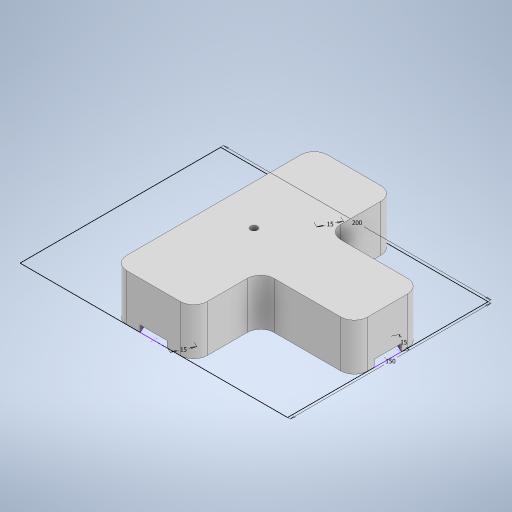
# Autodesk Inventor part: Area mv
Saved by Autodesk Inventor 2024 (Build 280153000, 153)
## iProperties
Created: 2024-03-01
Part Number: Area mv
Material: Generic
Document SubType Name: Modeling
Designer: laura
Density: 1 g/cm^3
Appearance: Default
Author: laura
Autodesk Inventor part; units mm, degrees
ref_plane "YZ Plane" through (0, 0, 0) normal (1, 0, 0) x (0, 1, 0)
ref_plane "XZ Plane" through (0, 0, 0) normal (0, 1, 0) x (-1, 0, 0)
ref_plane "XY Plane" through (0, 0, 0) normal (0, 0, 1) x (1, 0, 0)
sketch "Sketch1" plane through (0, 0, 0) normal (0, 1, 0) x (-1, 0, 0)
  line L0 (0, 0) -> (-200, 0)
  line L1 (-200, 0) -> (-200, -150)
  line L2 (-200, -150) -> (0, -150)
  line L3 (0, -150) -> (0, 0)
  line L4 (-109.8726, -150) -> (-90.1274, -150)
  line L5 (-200, -85.1274) -> (-200, -64.8726)
  line L6 (-186.0054, -60.2304) -> (-186.0054, -75)
  line L7 (-200, -64.8726) -> (-187.7125, -59.1428)
  arc A0 (-186.0054, -60.2304) -> (-187.7125, -59.1428) centre (-187.2054, -60.2304) ccw
  line L8 (-186.0054, -75) -> (-186.0054, -89.7696)
  line L9 (-199.8, -85) -> (-186.3697, -85) construction
  arc A1 (-187.7125, -90.8572) -> (-186.0054, -89.7696) centre (-187.2054, -89.7696) ccw
  line L10 (-187.7125, -90.8572) -> (-200, -85.1274)
  line L11 (-89.8726, -150) -> (-110.1274, -150)
  line L12 (-114.7696, -136.0054) -> (-100, -136.0054)
  line L13 (-110.1274, -150) -> (-115.8572, -137.7125)
  arc A2 (-114.7696, -136.0054) -> (-115.8572, -137.7125) centre (-114.7696, -137.2054) ccw
  line L14 (-100, -136.0054) -> (-85.2304, -136.0054)
  line L15 (-90, -149.8) -> (-90, -136.3697) construction
  arc A3 (-84.1428, -137.7125) -> (-85.2304, -136.0054) centre (-85.2304, -137.2054) ccw
  line L16 (-84.1428, -137.7125) -> (-89.8726, -150)
  line L17 (-90.1274, 0) -> (-109.8726, 0)
  line L18 (-85.2304, -13.9946) -> (-100, -13.9946)
  arc A4 (-115.8572, -12.2875) -> (-114.7696, -13.9946) centre (-114.7696, -12.7946) ccw
  arc A5 (-85.2304, -13.9946) -> (-84.1428, -12.2875) centre (-85.2304, -12.7946) ccw
  line L19 (-89.8726, 0) -> (-84.1428, -12.2875)
  line L20 (-110.1274, 0) -> (-89.8726, 0)
  line L21 (-110, -0.2) -> (-110, -13.6303) construction
  line L22 (-115.8572, -12.2875) -> (-110.1274, 0)
  line L23 (-100, -13.9946) -> (-114.7696, -13.9946)
  point P0 (-100, -150)
  point P1 (-100, -150)
  point P2 (-100, -150)
  point P3 (-100, -150)
  point P4 (-200, -75)
  point P5 (-186.2054, -91.3393)
  point P6 (-200, -75)
  point P7 (-200, -75)
  point P8 (-100, -150)
  point P9 (-83.6607, -136.2054)
  point P10 (-100, 0)
  point P11 (-116.3393, -13.7946)
  point P12 (-100, 0)
  point P13 (-100, 0)
  dimension "d0" = 200
  dimension "d1" = 150
  dimension "d2" = 15
  dimension "d13" = 15
  dimension "d14" = 15
  constraints: 48 end point, 12 point on circle, 8 midpoint, 6 centre point, 2 horizontal, 2 parallel, 1 perpendicular
  measures "d0" distance of L2.end L1.end
  measures "d1" distance of L1.end L0.end
  measures "d2" distance of L9.start point (-186.205, -91.339)
  measures "d13" distance of L15.start point (-83.661, -136.205)
  measures "d14" distance of L21.start point (-116.339, -13.795)
extrude "Extrusion1" add sketch "Sketch1" along normal blind 35
extrude "Extrusion2" cut sketch "Sketch1" along normal blind 5.2 contours L7 A0 L6 L8 A1 L10 L1
sketch "Sketch2" plane through (0, 35, 0) normal (0, 1, 0) x (1, 0, 0)
  line L0 (0, 150) -> (0, 0) projected
  line L1 (0, 75) -> (100, 75)
  circle A0 centre (100, 75) radius 2.6
  dimension "d9" = 100
  dimension "d10" = 5.2
  constraints: 2 end point, 1 centre point, 1 coincident, 1 horizontal, 1 midpoint
  measures "d9" distance of L1.start L1.end
  measures "d10" diameter of A0
extrude "Extrusion4" cut sketch "Sketch2" against normal blind 5.2
extrude "Extrusion5" cut sketch "Sketch1" along normal blind 4.8 contours L19 A5 L18 L23 A4 L22 L0 | L2 L13 A2 L12 L14 A3 L16
sketch "Sketch3" plane through (0, 0, 0) normal (0, -1, 0) x (1, 0, 0)
  line L0 (200, -150) -> (0, -150) projected
  line L1 (0, 0) -> (70, 0)
  line L2 (70, 0) -> (70, -150)
  line L3 (70, -150) -> (0, -150)
  line L4 (0, -150) -> (0, 0)
  line L5 (200, 0) -> (200, -64.8726) projected
  line L6 (200, 0) -> (130, 0)
  line L7 (130, 0) -> (130, -50)
  line L8 (130, -50) -> (200, -50)
  line L9 (200, -50) -> (200, 0)
  line L10 (200, -150) -> (130, -150)
  line L11 (130, -150) -> (130, -100)
  line L12 (130, -100) -> (200, -100)
  line L13 (200, -100) -> (200, -150)
  dimension "d17" = 70
  dimension "d18" = 70
  dimension "d19" = 50
  dimension "d20" = 70
  dimension "d21" = 50
  constraints: 24 end point, 6 parallel, 3 horizontal, 3 perpendicular, 3 point on line
  measures "d17" distance of L2.end L3.end
  measures "d18" distance of L8.end L7.end
  measures "d19" distance of L7.end L6.end
  measures "d20" distance of L11.end L12.end
  measures "d21" distance of L10.end L11.end
extrude "Extrusion6" cut sketch "Sketch3" against normal blind 40
fillet "Fillet1" radius 10 8 edges at (130, 17.5, -50) (200, 17.5, -50) (200, 17.5, -100) (130, 17.5, 0) (70, 17.5, 0) (70, 17.5, -150) (130, 17.5, -150) (130, 17.5, -100)
body "Solid1"
